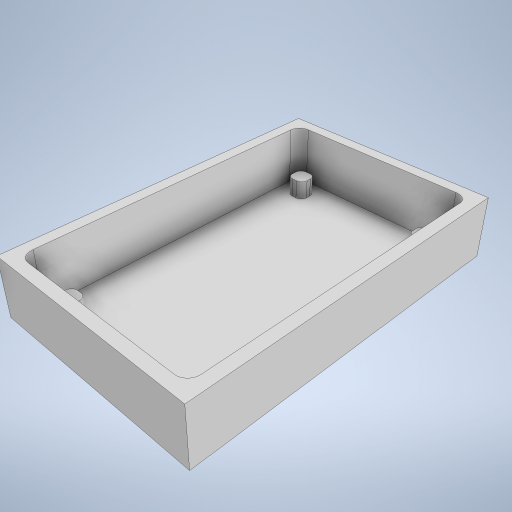
# Autodesk Inventor part: PrismGC
Saved by Autodesk Inventor 2024 (Build 280153000, 153)
## iProperties
Created: 2023-08-08
Part Number: PrismGC
Material: 常规
Document SubType Name: Modeling
Designer: liyuxuan
Density: 1 g/cm^3
Appearance: 默认
Author: liyuxuan
Autodesk Inventor part; units mm, degrees
ref_plane "YZ Plane" through (0, 0, 0) normal (1, 0, 0) x (0, 1, 0)
ref_plane "XZ Plane" through (0, 0, 0) normal (0, 1, 0) x (-1, 0, 0)
ref_plane "XY Plane" through (0, 0, 0) normal (0, 0, 1) x (1, 0, 0)
sketch "草图1" plane through (0, 0, 0) normal (0, 1, 0) x (-1, 0, 0)
  line L0 (0, 0) -> (-90, 0)
  line L1 (-90, 0) -> (-90, -140)
  line L2 (-90, -140) -> (0, -140)
  line L3 (0, -140) -> (0, 0)
  point P0 (-45, -70)
  dimension "d0" = 140
  dimension "d1" = 90
  constraints: 8 end point, 2 parallel, 1 horizontal, 1 perpendicular, 1 other
  measures "d0" distance of L0.end L1.end
  measures "d1" distance of L1.end L2.end
extrude "拉伸1" add sketch "草图1" along normal blind 25
sketch "草图2" plane through (0, 25, 0) normal (0, 1, 0) x (1, 0, 0)
  line L0 (90, 0) -> (90, 140) projected
  line L1 (90, 140) -> (0, 140) projected
  line L2 (0, 140) -> (0, 0) projected
  line L3 (0, 0) -> (90, 0) projected
  line L4 (5, 5) -> (85, 5)
  line L5 (85, 5) -> (85, 135)
  line L6 (85, 135) -> (5, 135)
  line L7 (5, 135) -> (5, 5)
  line L8 (5, 5) -> (85, 135) construction
  line L9 (85, 5) -> (5, 135) construction
  point P0 (45, 70)
  dimension "d4" = 80
  dimension "d5" = 130
  constraints: 12 end point, 2 midpoint, 2 parallel, 1 horizontal, 1 perpendicular
  measures "d4" distance of L6.end L5.end
  measures "d5" distance of L5.end L4.end
extrude "拉伸2" cut sketch "草图2" against normal blind 23.8 contours L7 L6 L5 L4
fillet "面圆角1" radius 5 1 edges at (5, 13.1, -5)
fillet "面圆角2" radius 5 1 edges at (5, 13.1, -135)
fillet "面圆角3" radius 5 1 edges at (85, 13.1, -135)
fillet "面圆角4" radius 5 1 edges at (85, 13.1, -5)
sketch "草图4" plane through (0, 1.2, 0) normal (0, 1, 0) x (1, 0, 0)
  arc A0 (80, 5) -> (85, 10) centre (80, 10) ccw projected
  line L0 (85, 130) -> (85, 10) projected
  arc A1 (85, 130) -> (80, 135) centre (80, 130) ccw projected
  line L1 (10, 135) -> (80, 135) projected
  arc A2 (10, 135) -> (5, 130) centre (10, 130) ccw projected
  line L2 (5, 10) -> (5, 130) projected
  arc A3 (5, 10) -> (10, 5) centre (10, 10) ccw projected
  line L3 (80, 5) -> (10, 5) projected
  line L4 (16.152, 18.12) -> (14.152, 18.12)
  line L5 (11.152, 15.12) -> (11.152, 13.12)
  line L6 (14.152, 10.12) -> (16.152, 10.12)
  line L7 (19.152, 13.12) -> (19.152, 15.12)
  line L8 (19.152, 18.12) -> (11.152, 10.12) construction
  line L9 (11.152, 18.12) -> (19.152, 10.12) construction
  arc A4 (11.152, 13.12) -> (14.152, 10.12) centre (14.152, 13.12) ccw
  arc A5 (16.152, 10.12) -> (19.152, 13.12) centre (16.152, 13.12) ccw
  arc A6 (19.152, 15.12) -> (16.152, 18.12) centre (16.152, 15.12) ccw
  arc A7 (14.152, 18.12) -> (11.152, 15.12) centre (14.152, 15.12) ccw
  line L10 (15.152, 14.12) -> (74.848, 14.12)
  line L11 (15.152, 14.12) -> (15.152, 125.88)
  line L12 (70.848, 15.12) -> (70.848, 13.12)
  arc A8 (70.848, 13.12) -> (73.848, 10.12) centre (73.848, 13.12) ccw
  line L13 (73.848, 10.12) -> (75.848, 10.12)
  arc A9 (75.848, 10.12) -> (78.848, 13.12) centre (75.848, 13.12) ccw
  line L14 (78.848, 13.12) -> (78.848, 15.12)
  arc A10 (78.848, 15.12) -> (75.848, 18.12) centre (75.848, 15.12) ccw
  line L15 (75.848, 18.12) -> (73.848, 18.12)
  arc A11 (73.848, 18.12) -> (70.848, 15.12) centre (73.848, 15.12) ccw
  line L16 (11.152, 126.88) -> (11.152, 124.88)
  arc A12 (11.152, 124.88) -> (14.152, 121.88) centre (14.152, 124.88) ccw
  line L17 (14.152, 121.88) -> (16.152, 121.88)
  arc A13 (16.152, 121.88) -> (19.152, 124.88) centre (16.152, 124.88) ccw
  line L18 (19.152, 124.88) -> (19.152, 126.88)
  arc A14 (19.152, 126.88) -> (16.152, 129.88) centre (16.152, 126.88) ccw
  line L19 (16.152, 129.88) -> (14.152, 129.88)
  arc A15 (14.152, 129.88) -> (11.152, 126.88) centre (14.152, 126.88) ccw
  line L20 (70.848, 126.88) -> (70.848, 124.88)
  arc A16 (70.848, 124.88) -> (73.848, 121.88) centre (73.848, 124.88) ccw
  line L21 (73.848, 121.88) -> (75.848, 121.88)
  arc A17 (75.848, 121.88) -> (78.848, 124.88) centre (75.848, 124.88) ccw
  line L22 (78.848, 124.88) -> (78.848, 126.88)
  arc A18 (78.848, 126.88) -> (75.848, 129.88) centre (75.848, 126.88) ccw
  line L23 (75.848, 129.88) -> (73.848, 129.88)
  arc A19 (73.848, 129.88) -> (70.848, 126.88) centre (73.848, 126.88) ccw
  point P0 (0, 0)
  point P1 (45, 70)
  point P2 (45, 70)
  point P3 (70.848, 10.12)
  point P4 (70.848, 18.12)
  point P5 (78.848, 10.12)
  point P6 (78.848, 18.12)
  point P7 (11.152, 121.88)
  point P8 (11.152, 129.88)
  point P9 (19.152, 121.88)
  point P10 (19.152, 129.88)
  point P11 (70.848, 121.88)
  point P12 (70.848, 129.88)
  point P13 (78.848, 121.88)
  point P14 (78.848, 129.88)
  dimension "d12" = 55.88
  dimension "d13" = 29.848
  dimension "d14" = 8
  dimension "d15" = 8
  dimension "d16" = 3
  dimension "d17" = 59.696
  dimension "d18" = 111.76
  dimension "d21" = 59.696
  dimension "d24" = 111.76
  constraints: 40 end point, 32 point on circle, 32 point on line, 16 centre point, 8 tangent, 3 equal radius, 3 horizontal, 2 midpoint, 2 parallel, 2 vertical, 1 coincident, 1 perpendicular, 73 other
  measures "d12" vertical distance of L10.start point (45, 70)
  measures "d13" horizontal distance of point (45, 70) L10.start
  measures "d14" distance of L9.end L8.end
  measures "d15" distance of L8.end L9.start
  measures "d16" radius of A4
  measures "d17" distance of L10.start L10.end
  measures "d18" distance of L10.start L11.end
  measures "d21" distance of L5.start L12.start
  measures "d24" distance of L5.start L16.start
extrude "拉伸3" add sketch "草图4" along normal blind 8 contours A6 L7 L10 L11 L4 | L11 L10 L7 A5 L6 A4 L5 A7 L4 | A11 L15 A10 L14 A9 L13 A8 L12 | A15 L19 A14 L18 A13 L17 A12 L16 | A19 L23 A18 L22 A17 L21 A16 L20
